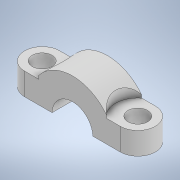
# Autodesk Inventor part: suction_clip_2_top
Saved by Autodesk Inventor 2022 (Build 260153000, 153)
## iProperties
Created: 2022-09-13
Part Number: suction_clip_2_top
Material: Generic
Document SubType Name: Modeling
Designer: dsdan
Density: 1 g/cm^3
Appearance: Default
Author: dsdan
Autodesk Inventor part; units mm, degrees
ref_plane "YZ Plane" through (0, 0, 0) normal (1, 0, 0) x (0, 1, 0)
ref_plane "XZ Plane" through (0, 0, 0) normal (0, 1, 0) x (-1, 0, 0)
ref_plane "XY Plane" through (0, 0, 0) normal (0, 0, 1) x (1, 0, 0)
sketch "Sketch1" plane through (0, 0, 0) normal (0, 0, 1) x (1, 0, 0)
  circle A0 centre (0, 0) radius 3.2
  line L0 (-3.1984, 0.1) -> (-10.25, 0.1)
  line L1 (-10.25, 0.1) -> (-10.25, 3.6)
  line L2 (-10.25, 3.6) -> (-5.6507, 3.6)
  arc A1 (5.6507, 3.6) -> (-5.6507, 3.6) centre (0, 0) ccw
  line L3 (5.6507, 3.6) -> (10.25, 3.6)
  line L4 (10.25, 3.6) -> (10.25, 2.7012)
  line L5 (10.25, 2.7012) -> (10.25, 0.1)
  line L6 (10.25, 0.1) -> (6.1992, 0.1)
  line L7 (6.1992, 0.1) -> (3.1984, 0.1)
  dimension "d0" = 6.4
  dimension "d1" = 0.1
  dimension "d2" = 3.5
  dimension "d3" = 3.5
  dimension "d4" = 10.25
  dimension "d5" = 10.25
  constraints: 16 end point, 4 point on circle, 3 horizontal, 2 centre point, 2 collinear, 2 perpendicular, 1 coincident, 1 point on line, 1 vertical
  measures "d0" diameter of A0
  measures "d1" distance from line of point (0, 0) L0
  measures "d2" distance of L0.end L1.end
  measures "d3" radial gap between concentric circles of A0 A1
  measures "d4" distance from line of point (0, 0) L1
  measures "d5" distance from line of point (0, 0) L5
extrude "Extrusion1" add sketch "Sketch1" along normal blind 5.5 contours A0 L0 L1 L2 A1 L3 L4 L5 L6 L7
sketch "Sketch2" plane through (-10.25, 3.6, 0) normal (0, 1, 0) x (1, 0, 0)
  circle A0 centre (2.75, -2.75) radius 3.5
  circle A1 centre (17.75, -2.75) radius 3.5
  line L0 (0, 0) -> (0, -5.5) projected
  line L1 (20.5, 0) -> (20.5, -5.5) projected
  point P0 (10.25, 0)
  point P1 (0, -2.75)
  dimension "d8" = 15
  dimension "d9" = 2.75
  dimension "d10" = 2.75
  dimension "d11" = 7
  constraints: 2 centre point, 2 horizontal alignment, 1 equal radius, 1 midpoint
  measures "d8" distance of A1.centre A0.centre
  measures "d9" distance from line of L0 A0.centre
  measures "d10" distance from line of L1 A1.centre
  measures "d11" diameter of A0
extrude "Extrusion2" cut sketch "Sketch2" along normal through all
sketch "Sketch3" plane through (-10.25, 3.6, 5.5) normal (0, 1, 0) x (1, 0, 0)
  arc A0 (4.9151, 0) -> (4.9151, 5.5) centre (2.75, 2.75) ccw projected
  circle A1 centre (2.75, 2.75) radius 1.55
  arc A2 (15.5849, 5.5) -> (15.5849, 0) centre (17.75, 2.75) ccw projected
  circle A3 centre (17.75, 2.75) radius 1.55
  line L0 (4.9151, 5.5) -> (15.5849, 5.5) projected
  line L1 (0, 5.5) -> (0, 0) projected
  line L2 (4.9151, 0) -> (0, 0) projected
  arc A4 (4.9151, 0) -> (4.9151, 5.5) centre (2.75, 2.75) ccw projected
  line L3 (4.9151, 5.5) -> (0, 5.5) projected
  line L4 (20.5, 5.5) -> (20.5, 0) projected
  line L5 (20.5, 5.5) -> (15.5849, 5.5) projected
  arc A5 (15.5849, 5.5) -> (15.5849, 0) centre (17.75, 2.75) ccw projected
  line L6 (20.5, 0) -> (15.5849, 0) projected
  circle A6 centre (17.75, 2.75) radius 2.75
  line L7 (20.5, 5.5) -> (15.5849, 5.5) projected
  circle A7 centre (2.75, 2.75) radius 2.75
  point P0 (10.25, 5.5)
  point P1 (15.5849, 0)
  point P2 (2.75, 0)
  point P3 (0, 2.75)
  point P4 (2.75, 5.5)
  point P5 (20.5, 2.75)
  point P6 (17.75, 0)
  point P7 (17.75, 5.5)
  dimension "d14" = 3.1
  constraints: 4 centre point, 4 coincident, 2 tangent, 1 equal radius
  measures "d14" diameter of A1
extrude "Extrusion3" cut sketch "Sketch3" against normal through all contours L2 L1 A7 | A7 L1 L3 | L5 L4 A6 | A6 L4 L6 | A1 | A3
equation "\"d3\" = d2"
equation "\"d5\" = d4"
equation "\"d9\" = d10"
body "Solid1"
